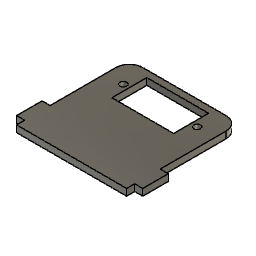
canon_A15_replacement (Autodesk Fusion 360 design; units mm, degrees)
Autodesk Fusion 360 part; units mm, degrees
sketch "Sketch1" plane through (0, 0, 0) normal (0, 0, 1) x (1, 0, 0)
  line L0 (0, 0) -> (40, 0)
  line L1 (40, 0) -> (40, 42)
  line L2 (40, 42) -> (0, 42)
  line L3 (0, 42) -> (0, 0)
  dimension "d1" = 40
  dimension "d2" = 42
  constraint horizontal L0
  constraint vertical L1
  constraint horizontal L2
  constraint vertical L3
  constraint coincident L0.start L3.end
  measures "d1" distance of L0.start L0.end
  measures "d2" distance of L0.start L2.end
extrude "Extrude1" add sketch "Sketch1" along normal blind 2.5
sketch "Sketch2" plane through (40, 0, 0) normal (1, 0, 0) x (0, 1, 0)
  line L0 (0, 0) -> (42, 0)
  line L1 (42, 0) -> (42, 2.5)
  line L2 (42, 2.5) -> (0, 2.5)
  line L3 (0, 2.5) -> (0, 0)
  line L4 (3, 2.5) -> (12.5, 2.5)
  line L5 (12.5, 2.5) -> (12.5, 0)
  line L6 (12.5, 0) -> (3, 0)
  line L7 (3, 0) -> (3, 2.5)
  dimension "d5" = 9.5
  dimension "d6" = 3
  constraint horizontal L4
  constraint vertical L5
  constraint horizontal L6
  constraint vertical L7
  constraint coincident L2 L4.start
  measures "d5" distance of L4.start L4.end
  measures "d6" distance of L3 L7
extrude "Extrude2" add sketch "Sketch2" along normal blind 3 contours L0 L2 L4 L5 L6 L7
sketch "Sketch3" plane through (0, 0, 0) normal (-1, 0, 0) x (0, -1, 0)
  line L0 (-42, 0) -> (0, 0)
  line L1 (0, 0) -> (0, 2.5)
  line L2 (0, 2.5) -> (-42, 2.5)
  line L3 (-42, 2.5) -> (-42, 0)
  line L4 (-3, 2.5) -> (-12.5, 2.5)
  line L5 (-12.5, 2.5) -> (-12.5, 0)
  line L6 (-12.5, 0) -> (-3, 0)
  line L7 (-3, 0) -> (-3, 2.5)
  dimension "d9" = 9.5
  dimension "d10" = 2.5
  dimension "d11" = 3
  constraint horizontal L4
  constraint vertical L5
  constraint horizontal L6
  constraint vertical L7
  constraint coincident L2 L4.start
  measures "d9" distance of L4.start L4.end
  measures "d10" distance of L4.start L6.end
  measures "d11" distance of L1 L7
extrude "Extrude3" add sketch "Sketch3" along normal blind 3 contours L0 L2 L4 L5 L6 L7
sketch "Sketch4" plane through (0, 0, 2.5) normal (0, 0, 1) x (-1, 0, 0)
  line L0 (0, -42) -> (0, -12.5)
  line L1 (0, -12.5) -> (3, -12.5)
  line L2 (3, -12.5) -> (3, -3)
  line L3 (3, -3) -> (0, -3)
  line L4 (0, -3) -> (0, 0)
  line L5 (0, 0) -> (-40, 0)
  line L6 (-40, 0) -> (-40, -3)
  line L7 (-40, -3) -> (-43, -3)
  line L8 (-43, -3) -> (-43, -12.5)
  line L9 (-43, -12.5) -> (-40, -12.5)
  line L10 (-40, -12.5) -> (-40, -42)
  line L11 (-40, -42) -> (0, -42)
  line L12 (-8.5, -39.5) -> (-31.5, -39.5)
  line L13 (-31.5, -39.5) -> (-31.5, -26.5)
  line L14 (-31.5, -26.5) -> (-8.5, -26.5)
  line L15 (-8.5, -26.5) -> (-8.5, -39.5)
  dimension "d14" = 23
  dimension "d15" = 13
  dimension "d16" = 8.5
  dimension "d17" = 14
  constraint horizontal L12
  constraint vertical L13
  constraint horizontal L14
  constraint vertical L15
  measures "d14" distance of L12.start L12.end
  measures "d15" distance of L12.start L14.end
  measures "d16" distance of L10 L13
  measures "d17" distance of L1 L14
extrude "Extrude4" cut sketch "Sketch4" against normal blind 3 contours L12 L13 L14 L15
sketch "Sketch5" plane through (0, 0, 2.5) normal (0, 0, 1) x (-1, 0, 0)
  line L0 (-31.5, -39.5) -> (-31.5, -26.5)
  line L1 (-31.5, -26.5) -> (-8.5, -26.5)
  line L2 (-8.5, -26.5) -> (-8.5, -39.5)
  line L3 (-8.5, -39.5) -> (-31.5, -39.5)
  line L4 (0, -42) -> (0, -12.5)
  line L5 (0, -12.5) -> (3, -12.5)
  line L6 (3, -12.5) -> (3, -3)
  line L7 (3, -3) -> (0, -3)
  line L8 (0, -3) -> (0, 0)
  line L9 (0, 0) -> (-40, 0)
  line L10 (-40, 0) -> (-40, -3)
  line L11 (-40, -3) -> (-43, -3)
  line L12 (-43, -3) -> (-43, -12.5)
  line L13 (-43, -12.5) -> (-40, -12.5)
  line L14 (-40, -12.5) -> (-40, -42)
  line L15 (-40, -42) -> (0, -42)
  circle A0 centre (-6.25, -33) radius 1.25
  dimension "d24" = 2.5
  dimension "d25" = 2.25
  dimension "d26" = 6.5
  measures "d24" diameter of A0
  measures "d25" distance of L2 A0.centre
  measures "d26" distance of L1 A0.centre
extrude "Extrude5" cut sketch "Sketch5" against normal blind 3 contours A0
sketch "Sketch6" plane through (0, 0, 2.5) normal (0, 0, 1) x (-1, 0, 0)
  circle A0 centre (-6.25, -33) radius 1.25
  line L0 (-31.5, -39.5) -> (-31.5, -26.5)
  line L1 (-31.5, -26.5) -> (-8.5, -26.5)
  line L2 (-8.5, -26.5) -> (-8.5, -39.5)
  line L3 (-8.5, -39.5) -> (-31.5, -39.5)
  line L4 (0, -42) -> (0, -12.5)
  line L5 (0, -12.5) -> (3, -12.5)
  line L6 (3, -12.5) -> (3, -3)
  line L7 (3, -3) -> (0, -3)
  line L8 (0, -3) -> (0, 0)
  line L9 (0, 0) -> (-40, 0)
  line L10 (-40, 0) -> (-40, -3)
  line L11 (-40, -3) -> (-43, -3)
  line L12 (-43, -3) -> (-43, -12.5)
  line L13 (-43, -12.5) -> (-40, -12.5)
  line L14 (-40, -12.5) -> (-40, -42)
  line L15 (-40, -42) -> (0, -42)
  circle A1 centre (-33.75, -33) radius 1.25
  dimension "d29" = 2.5
  dimension "d30" = 2.25
  dimension "d31" = 6.5
  measures "d29" diameter of A1
  measures "d30" distance of L0 A1.centre
  measures "d31" distance of L1 A1.centre
extrude "Extrude6" cut sketch "Sketch6" against normal blind 3 contours A1
extrude "Extrude7" add 1 faces at (40, 22.3333, 0.8333) along direction (1, 0, 0) blind 0.5
extrude "Extrude8" add 1 faces at (40, 2, 1.6667) along direction (1, 0, 0) blind 0.5
extrude "Extrude9" add 1 faces at (0, 32.1667, 0.8333) along direction (-1, 0, 0) blind 0.5
extrude "Extrude10" add 1 faces at (0, 1, 1.6667) along direction (-1, 0, 0) blind 0.5
extrude "Extrude11" add 1 faces at (-3, 9.3333, 1.6667) along direction (-1, 0, 0) blind 0.5
extrude "Extrude12" add 1 faces at (43, 6.1667, 1.6667) along direction (1, 0, 0) blind 0.5
fillet "Fillet3" radius 5 1 edges at (-0.5, 42, 1.25)
fillet "Fillet4" radius 5 1 edges at (40.5, 42, 1.25)
